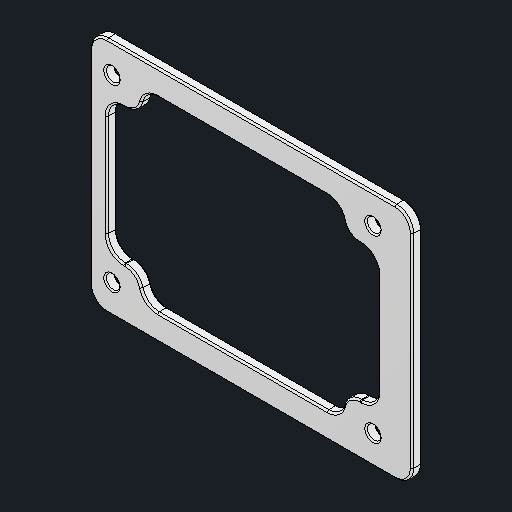
# Autodesk Inventor part: temp-logger-base-plate-v2
Saved by Autodesk Inventor 2027.1 (Build 311270010, 270A)
## iProperties
Created: 2025-07-16
Part Number: temp-logger-base-plate-v2
Material: ABS Plastic
Document SubType Name: Modeling
Designer: kuzmin
Density: 1.06 g/cm^3
Appearance: Smooth - White
Author: kuzmin
Autodesk Inventor part; units mm, degrees
ref_plane "YZ Plane" through (0, 0, 0) normal (1, 0, 0) x (0, 1, 0)
ref_plane "XZ Plane" through (0, 0, 0) normal (0, 1, 0) x (-1, 0, 0)
ref_plane "XY Plane" through (0, 0, 0) normal (0, 0, 1) x (1, 0, 0)
sketch "Sketch1" plane through (0, 0, 0) normal (0, 0, 1) x (1, 0, 0)
  line L0 (-45, 35) -> (50, 35)
  line L1 (50, 35) -> (50, -35)
  line L2 (50, -35) -> (-45, -35)
  line L3 (-45, -35) -> (-45, 35)
  line L4 (-38.5, 26.5) -> (38.5, 26.5) construction
  line L5 (38.5, 26.5) -> (38.5, -26.5) construction
  line L6 (38.5, -26.5) -> (-38.5, -26.5) construction
  line L7 (-38.5, -26.5) -> (-38.5, 26.5) construction
  circle A0 centre (-38.5, 26.5) radius 2.5
  circle A1 centre (38.5, 26.5) radius 2.5
  circle A2 centre (38.5, -26.5) radius 2.5
  circle A3 centre (-38.5, -26.5) radius 2.5
  line L8 (-30, 27.5) -> (30, 27.5)
  line L9 (30, 27.5) -> (30, -27.5)
  line L10 (30, -27.5) -> (-30, -27.5)
  line L11 (-30, -27.5) -> (-30, 27.5)
  line L12 (30, 20) -> (40, 20)
  line L13 (40, 20) -> (40, -20)
  line L14 (40, -20) -> (30, -20)
  line L15 (30, -20) -> (30, 20)
  line L16 (-30, 20) -> (-40, 20)
  line L17 (-40, 20) -> (-40, -20)
  line L18 (-40, -20) -> (-30, -20)
  line L19 (-30, -20) -> (-30, 20)
  point P0 (0, 0)
  point P1 (50, 0)
  point P2 (2.5, 35)
  point P3 (38.5, 0)
  point P4 (0, 26.5)
  point P5 (30, 0)
  point P6 (0, 27.5)
  point P7 (-40, 0)
  point P8 (40, 0)
  point P9 (30, -20)
  dimension "d1" = 70
  dimension "d2" = 77
  dimension "d3" = 53
  dimension "d14" = 5
  dimension "d23" = 45
  dimension "d24" = 50
  dimension "d25" = 55
  dimension "d26" = 60
  dimension "d27" = 40
  dimension "d28" = 10
  dimension "d29" = 10
  constraints: 40 end point, 11 parallel, 8 coincident, 8 midpoint, 5 horizontal, 5 horizontal alignment, 5 perpendicular, 4 centre point, 3 equal radius, 2 point on line, 2 vertical alignment
  measures "d1" distance of L0.end L1.end
  measures "d2" distance of L4.start L4.end
  measures "d3" distance of L4.end L5.end
  measures "d14" diameter of A0
  measures "d23" distance from line of L3 point (0, 0)
  measures "d24" distance from line of L1 point (0, 0)
  measures "d25" distance of L8.end L9.end
  measures "d26" distance of L8.start L8.end
  measures "d27" distance of L16.end L17.end
  measures "d28" distance of L16.start L16.end
  measures "d29" distance of L12.start L12.end
extrude "Extrusion1" add sketch "Sketch1" along normal blind 3 contours L0 L1 L2 L3 | A0 | A1 | A2 | A3
hole "Hole1" at (38.5, 26.5, 0) at (38.5, -26.5, 0) at (-38.5, -26.5, 0) at (-38.5, 26.5, 0) direction (0, 0, 1) diameter 4 end through all
fillet "Fillet1" radius 5 16 edges at (50, 35, 1.5) (50, -35, 1.5) (-45, -35, 1.5) (-45, 35, 1.5) (-30, 27.5, 1.5) (30, 27.5, 1.5) (30, -27.5, 1.5) (-30, -27.5, 1.5) (-30, 20, 1.5) (-40, 20, 1.5) (-40, -20, 1.5) (-30, -20, 1.5) (30, 20, 1.5) (40, 20, 1.5) (40, -20, 1.5) (30, -20, 1.5)
chamfer "Chamfer2" distance 0.5 angle 45 48 edges at (2.5, 35, 0) (-43.5355, 33.5355, 0) (-45, 0, 0) (-43.5355, -33.5355, 0) (2.5, -35, 0) (48.5355, -33.5355, 0) (50, 0, 0) (48.5355, 33.5355, 0) (2.5, 35, 3) (-43.5355, 33.5355, 3) (-45, 0, 3) (-43.5355, -33.5355, 3) (2.5, -35, 3) (48.5355, -33.5355, 3) (50, 0, 3) (48.5355, 33.5355, 3) (0, 27.5, 3) (28.0619, 26.4528, 3) (31.6206, 21.0472, 3) (38.5355, 18.5355, 3) (40, 0, 3) (38.5355, -18.5355, 3) (31.6206, -21.0472, 3) (28.0619, -26.4528, 3) (0, -27.5, 3) (-28.0619, -26.4528, 3) (-31.6206, -21.0472, 3) (-38.5355, -18.5355, 3) (-40, 0, 3) (-38.5355, 18.5355, 3) (-31.6206, 21.0472, 3) (-28.0619, 26.4528, 3) (0, 27.5, 0) (28.0619, 26.4528, 0) (31.6206, 21.0472, 0) (38.5355, 18.5355, 0) (40, 0, 0) (38.5355, -18.5355, 0) (31.6206, -21.0472, 0) (28.0619, -26.4528, 0) (0, -27.5, 0) (-28.0619, -26.4528, 0) (-31.6206, -21.0472, 0) (-38.5355, -18.5355, 0) (-40, 0, 0) (-38.5355, 18.5355, 0) (-31.6206, 21.0472, 0) (-28.0619, 26.4528, 0)
chamfer "Chamfer3" distance 0.4 angle 45 8 edges at (-38.5, 24.5, 3) (-38.5, -28.5, 3) (38.5, 24.5, 3) (38.5, -28.5, 3) (-38.5, 24.5, 0) (38.5, 24.5, 0) (38.5, -28.5, 0) (-38.5, -28.5, 0)
equation "\"d1\" = width"
equation "\"d23\" = 0.5 * length"
equation "\"d4\" = thickness"
equation "\"width\" = 70"
equation "\"thickness\" = 3"
equation "\"bump\" = 3"
equation "\"length\" = 90"
body "Solid1"
